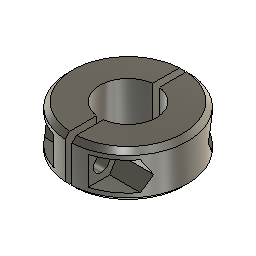
Dual Shaft Shredder (Autodesk Fusion 360 archive; units mm, degrees)
design "Double-Split Shaft Collars (20x20)"
Autodesk Fusion 360 part; units mm, degrees
sketch "Sketch1" plane through (0, 0, 0) normal (0, 0, 1) x (1, 0, 0)
  circle A0 centre (0, 0) radius 6
  circle A1 centre (0, 0) radius 13
  circle A2 centre (0, 0) radius 6.15
  line L0 (0.75, 20) -> (-0.75, 20)
  line L1 (-0.75, 20) -> (-0.75, -20)
  line L2 (-0.75, -20) -> (0.75, -20)
  line L3 (0.75, -20) -> (0.75, 20)
  line L4 (0.75, 20) -> (-0.75, -20) construction
  line L5 (-0.75, 20) -> (0.75, -20) construction
  line L6 (0.75, -9.336) -> (-0.75, -9.336)
  line L7 (0, -6.15) -> (0, -13)
  point P0 (0, -6.15)
  point P1 (0, -13)
  dimension "d1" = 12
  dimension "d2" = 0.15
  dimension "d5" = 1.5
  dimension "d7" = 26
  dimension "d44" = 3.186
  dimension "d45" = 40
  dimension "d46" = 6.85
  constraint coincident A0.centre A1.centre
  constraint concentric A0 A1
  constraint horizontal L0
  constraint perpendicular L0 L1
  constraint parallel L0 L2
  constraint parallel L1 L3
  constraint coincident L4 A0.centre
  constraint coincident L5 A0.centre
  constraint coincident L3 L6.start
  constraint coincident L1 L6.end
  constraint perpendicular L1 L6
  constraint coincident A2 P0
  constraint coincident A1 P1
  constraint coincident P0 L7.start
  constraint coincident P1 L7.end
  constraint parallel L3 L7
  measures "d1" diameter of A0
  measures "d5" distance of L1.end L2.end
  measures "d7" diameter of A1
  measures "d44" distance of L6 P0
  measures "d45" vertical distance of L0.end L2.end
  measures "d46" distance of P0 P1
extrude "Extrude1" add sketch "Sketch1" along normal blind 10 contours A1 A2 L3 | A1 A2 L1 makes body 1 at (8.6713, -9.6855, 6.6667) makes body 2 at (-7.1905, -10.8304, 3.3333)
sketch "Sketch2" plane through (-0.75, 0, 0) normal (1, 0, 0) x (0, 1, 0)
  line L0 (6.1041, 0) -> (12.9783, 0)
  line L1 (12.9783, 0) -> (12.9783, 10)
  line L2 (12.9783, 10) -> (6.1041, 10)
  line L3 (6.1041, 10) -> (6.1041, 0)
  line L4 (7.7514, 8.1) -> (5.9617, 5)
  line L5 (5.9617, 5) -> (7.7514, 1.9)
  line L6 (7.7514, 1.9) -> (11.331, 1.9)
  line L7 (11.331, 1.9) -> (13.1208, 5)
  line L8 (13.1208, 5) -> (11.331, 8.1)
  line L9 (11.331, 8.1) -> (7.7514, 8.1)
  circle A0 centre (9.5412, 5) radius 1.75
  line L10 (9.5412, 5) -> (6.1041, 5) construction
  line L11 (9.5412, 5) -> (12.9783, 5) construction
  line L12 (9.5412, 5) -> (9.5412, 0) construction
  line L13 (9.5412, 5) -> (9.5412, 10) construction
  line L14 (11.331, 8.1) -> (12.9783, 8.1)
  line L15 (11.331, 1.9) -> (12.9783, 1.9)
  line L16 (0, 0) -> (0, 10)
  line L17 (-9.5412, 5) -> (-9.5412, 10) construction
  line L18 (-12.9783, 0) -> (-12.9783, 10)
  line L19 (-9.5412, 5) -> (-12.9783, 5) construction
  line L20 (-11.331, 1.9) -> (-13.1208, 5)
  line L21 (-11.331, 8.1) -> (-12.9783, 8.1)
  line L22 (-7.7514, 1.9) -> (-11.331, 1.9)
  line L23 (-6.1041, 10) -> (-6.1041, 0)
  line L24 (-11.331, 1.9) -> (-12.9783, 1.9)
  circle A1 centre (-9.5412, 5) radius 1.75
  line L25 (-9.5412, 5) -> (-9.5412, 0) construction
  line L26 (-9.5412, 5) -> (-6.1041, 5) construction
  line L27 (-5.9617, 5) -> (-7.7514, 1.9)
  line L28 (-13.1208, 5) -> (-11.331, 8.1)
  line L29 (-11.331, 8.1) -> (-7.7514, 8.1)
  line L30 (-7.7514, 8.1) -> (-5.9617, 5)
  point P0 (9.5412, 5)
  point P1 (-9.5412, 5)
  dimension "d17" = 3.1
  dimension "d18" = 3.5
  constraint coincident P0 A0.centre
  constraint midpoint L3 L10.end
  constraint midpoint L1 L11.end
  constraint coincident L0 L12.end
  constraint perpendicular L0 L12
  constraint coincident L2 L13.end
  constraint perpendicular L2 L13
  constraint equal L10 L11
  constraint coincident L1 L14.end
  constraint perpendicular L1 L14
  constraint coincident L1 L15.end
  constraint perpendicular L1 L15
  constraint horizontal L10
  constraint coincident L16.start origin
  constraint vertical L16
  constraint horizontal L9
  constraint symmetric L0.start L16 L23.end
  constraint symmetric L0.end L16 L18.start
  constraint symmetric L1.end L16 L18.end
  constraint symmetric L2.end L16 L23.start
  constraint symmetric L4.start L16 L29.end
  constraint symmetric L4.end L16 L27.start
  constraint symmetric L5.end L16 L22.start
  constraint symmetric L6.end L16 L20.start
  constraint symmetric L7.end L16 L20.end
  constraint symmetric L8.end L16 L21.start
  constraint symmetric P0 L16 P1
  constraint symmetric A0 L16 A1
  constraint symmetric L10.end L16 L26.end
  constraint symmetric L11.end L16 L19.end
  constraint symmetric L12.end L16 L25.end
  constraint symmetric L13.end L16 L17.end
  constraint symmetric L14.end L16 L21.end
  constraint symmetric L15.end L16 L24.end
  measures "d17" distance of P0 L9
  measures "d18" diameter of A0
extrude "Extrude2" cut sketch "Sketch2" along normal mid plane 200 contours A0 | A1 bodies 1 2
extrude "Extrude3" cut sketch "Sketch2" against normal blind 10 from surface at -3 contours L3 L4 L5 | L1 L3 L4 L5 L6 L7 L8 L9 | L1 L7 L15 | L1 L8 L14 | A0 | L18 L20 L24 | L18 L20 L28 | L18 L20 L22 L23 L27 L28 L29 L30 | L18 L21 L28 | L23 L27 L30 | A1 bodies 2
extrude "Extrude4" cut sketch "Sketch2" along normal blind 100 from surface at 4.5 contours L3 L4 L5 | L1 L3 L4 L5 L6 L7 L8 L9 | L1 L7 L15 | L1 L8 L14 | L18 L20 L24 | L18 L20 L28 | L18 L20 L22 L23 L27 L28 L29 L30 | L18 L21 L28 | L23 L27 L30 | A1 bodies 1
chamfer "Chamfer1" distance 1 angle 45 4 edges at (13, 0, 0) (-13, 0, 0) (13, 0, 10) (-13, 0, 10) on bodies 1 2
ref_plane "WorkPlane1" through (0, -16, 0) normal (0, 1, 0) x (0, 0, 1)
sketch "Sketch3" plane through (0, -16, 0) normal (0, 1, 0) x (1, 0, 0)
  line L0 (2.7682, -5.085) -> (2.7681, -3.3241)
  spline S0 degree 5 poles (0.7027, -4.5337) (0.7103, -4.5353) (0.7255, -4.5381) (0.7483, -4.5414) (0.7791, -4.5438) (0.8177, -4.5436) (0.8566, -4.5399) (0.8955, -4.5325) (0.9341, -4.5209) (0.9719, -4.5044) (1.0082, -4.4824) (1.0425, -4.4542) (1.0739, -4.4193) (1.1016, -4.3775) (1.125, -4.3289) (1.1434, -4.274) (1.1562, -4.2138) (1.1629, -4.1493) (1.1634, -4.0822) (1.1577, -4.0144) (1.146, -3.9481) (1.1285, -3.8854) (1.1057, -3.8281) (1.0777, -3.7778) (1.0448, -3.7354) (1.0072, -3.7014) (0.9735, -3.681) (0.9462, -3.6696) (0.9271, -3.6638) (0.9173, -3.6613) knots 0 0 0 0 0 0 0.04 0.08 0.12 0.16 0.2 0.24 0.28 0.32 0.36 0.4 0.44 0.48 0.52 0.56 0.6 0.64 0.68 0.72 0.76 0.8 0.84 0.88 0.92 0.96 1 1 1 1 1 1
  line L1 (-3.1848, -3.0239) -> (-0.2225, -1.1432)
  arc A0 (0.0476, -6.9119) -> (-0.0024, -6.8619) centre (0.0476, -6.8619) cw
  line L2 (-1.3972, -3.7392) -> (-1.0488, -3.7773)
  line L3 (-1.627, -6.2849) -> (0.0512, -7.3504)
  line L4 (0.0476, -6.3678) -> (0.924, -6.3678)
  line L5 (1.6752, -6.3065) -> (0.8223, -5.3819)
  line L6 (3.2854, -7.1282) -> (0.0564, -9.2039)
  line L7 (-1.6303, -4.4396) -> (-1.102, -4.3813)
  line L8 (-0.0261, -5.4201) -> (-0.0261, -5.3437)
  line L9 (3.2854, -5.085) -> (3.2854, -7.1282)
  line L10 (0.0632, -3.9467) -> (0.0632, -4.4154)
  spline S1 degree 5 poles (1.7234, -4.437) (1.723, -4.4408) (1.722, -4.4487) (1.7198, -4.4614) (1.7155, -4.4798) (1.7078, -4.5055) (1.6978, -4.5337) (1.6855, -4.5642) (1.6713, -4.5965) (1.6556, -4.6296) (1.6392, -4.6624) (1.6226, -4.6937) (1.6066, -4.7223) (1.5916, -4.7474) (1.5781, -4.7684) (1.5661, -4.7851) (1.5578, -4.7951) (1.5523, -4.8006) (1.5489, -4.8035) (1.5473, -4.8047) knots 0 0 0 0 0 0 0.066667 0.133333 0.2 0.266667 0.333333 0.4 0.466667 0.533333 0.6 0.666667 0.733333 0.8 0.866667 0.933333 1 1 1 1 1 1
  line L11 (-1.0788, -5.1426) -> (-1.1684, -4.8048)
  line L12 (-2.6786, -5.0947) -> (-2.6686, -6.8612)
  line L13 (0.1369, -4.8048) -> (1.7234, -4.8047)
  line L14 (-2.6692, -3.3091) -> (0.0547, -1.5798)
  line L15 (-0.6159, -5.5515) -> (-1.0229, -5.5515)
  line L16 (-1.6325, -5.3094) -> (-1.2801, -6.5052)
  line L17 (0.1369, -4.8048) -> (-0.4862, -4.8048)
  line L18 (1.7234, -5.0851) -> (1.7234, -3.8946)
  line L19 (0.7027, -4.5337) -> (0.7027, -3.6651)
  line L20 (0.8223, -5.3819) -> (1.7234, -5.3819)
  line L21 (-1.6274, -3.8853) -> (0.0512, -2.8196)
  line L22 (3.2854, -5.085) -> (3.2853, -3.0418)
  line L23 (-3.1957, -5.0948) -> (-3.1848, -3.0239)
  line L24 (1.7234, -5.0851) -> (1.7234, -6.2754)
  line L25 (2.7682, -5.085) -> (2.7682, -6.8459)
  line L26 (-1.6338, -5.0945) -> (-1.627, -6.2849)
  line L27 (0.9173, -3.6613) -> (0.7027, -3.6651)
  line L28 (-0.6538, -6.9028) -> (-0.5276, -6.9028)
  line L29 (0.924, -6.3678) -> (-0.0261, -5.4201)
  line L30 (-0.2225, -1.1432) -> (0.0565, -0.9661)
  arc A1 (-0.0024, -6.4178) -> (0.0476, -6.3678) centre (0.0476, -6.4178) cw
  spline S2 degree 5 poles (-1.102, -4.3813) (-1.0994, -4.3879) (-1.094, -4.4007) (-1.0852, -4.4189) (-1.0722, -4.4412) (-1.0536, -4.4657) (-1.0329, -4.4869) (-1.0102, -4.505) (-0.9858, -4.5202) (-0.9601, -4.5327) (-0.9337, -4.543) (-0.9072, -4.5513) (-0.8808, -4.5579) (-0.8548, -4.5628) (-0.8291, -4.5657) (-0.8032, -4.5659) (-0.7769, -4.563) (-0.7501, -4.5564) (-0.7232, -4.546) (-0.6972, -4.532) (-0.6737, -4.5148) (-0.6542, -4.4953) (-0.6398, -4.4745) (-0.6311, -4.4533) (-0.6271, -4.4326) (-0.6266, -4.4132) (-0.6278, -4.3955) (-0.6292, -4.3796) (-0.6305, -4.365) (-0.6326, -4.3504) (-0.6371, -4.3345) (-0.6459, -4.3162) (-0.6606, -4.2952) (-0.6818, -4.2721) (-0.709, -4.2489) (-0.7408, -4.228) (-0.7756, -4.2116) (-0.8113, -4.2014) (-0.8463, -4.1978) (-0.8792, -4.1992) (-0.909, -4.2032) (-0.935, -4.2065) (-0.9567, -4.2059) (-0.9737, -4.1984) (-0.9858, -4.1823) (-0.993, -4.1564) (-0.9948, -4.1275) (-0.9938, -4.1011) (-0.9922, -4.0814) (-0.9911, -4.071) knots 0 0 0 0 0 0 0.022222 0.044444 0.066667 0.088889 0.111111 0.133333 0.155556 0.177778 0.2 0.222222 0.244444 0.266667 0.288889 0.311111 0.333333 0.355556 0.377778 0.4 0.422222 0.444444 0.466667 0.488889 0.511111 0.533333 0.555556 0.577778 0.6 0.622222 0.644444 0.666667 0.688889 0.711111 0.733333 0.755556 0.777778 0.8 0.822222 0.844444 0.866667 0.888889 0.911111 0.933333 0.955556 0.977778 1 1 1 1 1 1
  line L31 (-0.4893, -6.8744) -> (0.1369, -4.8048)
  line L32 (-1.1684, -4.8048) -> (-1.6322, -4.8024)
  line L33 (-3.1842, -7.1465) -> (0.0564, -9.2039)
  line L34 (-3.1957, -5.0948) -> (-3.1842, -7.1465)
  spline S3 degree 5 poles (-1.0488, -3.7773) (-1.0435, -3.768) (-1.0328, -3.75) (-1.0169, -3.7246) (-0.9961, -3.6939) (-0.9705, -3.6606) (-0.9455, -3.6323) (-0.921, -3.609) (-0.8972, -3.5902) (-0.874, -3.5754) (-0.8515, -3.564) (-0.8299, -3.5552) (-0.8091, -3.5484) (-0.7889, -3.543) (-0.7692, -3.539) (-0.7495, -3.5365) (-0.7293, -3.536) (-0.7084, -3.5381) (-0.6864, -3.5433) (-0.6638, -3.5517) (-0.641, -3.5634) (-0.6188, -3.5783) (-0.5981, -3.5958) (-0.5797, -3.6156) (-0.5642, -3.6371) (-0.5522, -3.6597) (-0.5437, -3.683) (-0.5388, -3.7065) (-0.5376, -3.7299) (-0.5398, -3.7531) (-0.5452, -3.7759) (-0.5537, -3.7985) (-0.5651, -3.8207) (-0.5794, -3.8423) (-0.5968, -3.8625) (-0.6177, -3.8805) (-0.6424, -3.8953) (-0.6709, -3.9061) (-0.703, -3.9124) (-0.7379, -3.9144) (-0.7745, -3.9129) (-0.8112, -3.9092) (-0.8463, -3.9046) (-0.8785, -3.9005) (-0.9065, -3.8982) (-0.9299, -3.8982) (-0.9484, -3.9012) (-0.9622, -3.9071) (-0.9719, -3.9159) (-0.9782, -3.9273) (-0.9818, -3.9409) (-0.9837, -3.9564) (-0.9846, -3.9734) (-0.9851, -3.9914) (-0.9858, -4.0103) (-0.987, -4.0299) (-0.9883, -4.046) (-0.9896, -4.0584) (-0.9906, -4.0668) (-0.9911, -4.071) knots 0 0 0 0 0 0 0.018182 0.036364 0.054545 0.072727 0.090909 0.109091 0.127273 0.145455 0.163636 0.181818 0.2 0.218182 0.236364 0.254545 0.272727 0.290909 0.309091 0.327273 0.345455 0.363636 0.381818 0.4 0.418182 0.436364 0.454545 0.472727 0.490909 0.509091 0.527273 0.545455 0.563636 0.581818 0.6 0.618182 0.636364 0.654545 0.672727 0.690909 0.709091 0.727273 0.745455 0.763636 0.781818 0.8 0.818182 0.836364 0.854545 0.872727 0.890909 0.909091 0.927273 0.945455 0.963636 0.981818 1 1 1 1 1 1
  line L35 (1.7234, -6.2754) -> (0.0512, -7.3504)
  line L36 (-0.5884, -5.1425) -> (-1.0788, -5.1426)
  line L37 (-0.0024, -6.8619) -> (-0.0024, -6.4178)
  line L38 (2.7681, -3.3241) -> (0.0547, -1.5798)
  line L39 (3.2853, -3.0418) -> (0.3344, -1.1447)
  line L40 (1.7234, -3.8946) -> (0.0512, -2.8196)
  line L41 (-1.0229, -5.5515) -> (-0.8136, -6.2122)
  line L42 (0.5197, -3.1208) -> (0.037, -3.1208)
  line L43 (-2.6686, -6.8612) -> (0.0547, -8.5903)
  arc A2 (-0.4893, -6.8744) -> (-0.5276, -6.9028) centre (-0.5276, -6.8628) cw
  line L44 (-0.8136, -6.2122) -> (-0.6159, -5.5515)
  line L45 (0.7334, -6.9119) -> (0.0476, -6.9119)
  spline S4 degree 5 poles (-0.1624, -4.0774) (-0.1492, -4.0711) (-0.1239, -4.0591) (-0.0895, -4.0426) (-0.0509, -4.024) (-0.0144, -4.006) (0.011, -3.9928) (0.0268, -3.9837) (0.0356, -3.9772) (0.0414, -3.9711) (0.0483, -3.9628) (0.0601, -3.9498) (0.0783, -3.9301) (0.1019, -3.9027) (0.1273, -3.8674) (0.1499, -3.8248) (0.1656, -3.7763) (0.1713, -3.7233) (0.1667, -3.6681) (0.1535, -3.6125) (0.1348, -3.5589) (0.1137, -3.5087) (0.0929, -3.4635) (0.0733, -3.4236) (0.054, -3.3889) (0.0332, -3.3585) (0.0084, -3.3317) (-0.0223, -3.3073) (-0.0597, -3.2848) (-0.1033, -3.264) (-0.1518, -3.2447) (-0.2034, -3.2271) (-0.2561, -3.2114) (-0.3084, -3.1979) (-0.3592, -3.1867) (-0.4078, -3.1778) (-0.4448, -3.1726) (-0.4714, -3.1697) (-0.4886, -3.1683) (-0.4971, -3.1677) knots 0 0 0 0 0 0 0.028571 0.057143 0.085714 0.114286 0.142857 0.171429 0.2 0.228571 0.257143 0.285714 0.314286 0.342857 0.371429 0.4 0.428571 0.457143 0.485714 0.514286 0.542857 0.571429 0.6 0.628571 0.657143 0.685714 0.714286 0.742857 0.771429 0.8 0.828571 0.857143 0.885714 0.914286 0.942857 0.971429 1 1 1 1 1 1
  line L46 (2.7682, -6.8459) -> (0.0547, -8.5903)
  line L47 (0.0565, -0.9661) -> (0.3344, -1.1447)
  line L48 (-1.6338, -5.0945) -> (-1.6274, -3.8853)
  spline S5 degree 5 poles (-1.6746, -4.5564) (-1.6709, -4.5624) (-1.6629, -4.5744) (-1.6495, -4.5925) (-1.6286, -4.6166) (-1.5972, -4.6469) (-1.5606, -4.6773) (-1.5183, -4.7076) (-1.4702, -4.7375) (-1.4155, -4.7669) (-1.3538, -4.7953) (-1.2849, -4.8222) (-1.2087, -4.847) (-1.126, -4.8691) (-1.0378, -4.8878) (-0.9462, -4.9022) (-0.853, -4.9117) (-0.7605, -4.9159) (-0.6708, -4.9147) (-0.5857, -4.9082) (-0.5062, -4.8971) (-0.4333, -4.8826) (-0.3669, -4.8657) (-0.3072, -4.8476) (-0.2535, -4.8291) (-0.2052, -4.8104) (-0.1614, -4.7908) (-0.1214, -4.7696) (-0.0844, -4.7456) (-0.0501, -4.7179) (-0.0187, -4.686) (0.009, -4.6503) (0.0322, -4.6112) (0.05, -4.5697) (0.0617, -4.5269) (0.0672, -4.4837) (0.067, -4.4409) (0.0618, -4.3993) (0.0526, -4.3595) (0.04, -4.3217) (0.0244, -4.286) (0.006, -4.2522) (-0.015, -4.2201) (-0.0388, -4.1894) (-0.0654, -4.1598) (-0.0947, -4.1313) (-0.1204, -4.1093) (-0.1409, -4.0932) (-0.1552, -4.0826) (-0.1624, -4.0774) knots 0 0 0 0 0 0 0.022222 0.044444 0.066667 0.088889 0.111111 0.133333 0.155556 0.177778 0.2 0.222222 0.244444 0.266667 0.288889 0.311111 0.333333 0.355556 0.377778 0.4 0.422222 0.444444 0.466667 0.488889 0.511111 0.533333 0.555556 0.577778 0.6 0.622222 0.644444 0.666667 0.688889 0.711111 0.733333 0.755556 0.777778 0.8 0.822222 0.844444 0.866667 0.888889 0.911111 0.933333 0.955556 0.977778 1 1 1 1 1 1
  line L49 (-2.6786, -5.0947) -> (-2.6692, -3.3091)
  line L50 (0.0527, -4.5564) -> (0.0527, -4.8048)
  line L51 (0.037, -3.1208) -> (0.037, -3.368)
  line L52 (-0.4862, -4.8048) -> (-0.5884, -5.1425)
  point P0 (-0.5387, -3.7178)
  point P1 (-0.5891, -3.606)
  point P2 (0.8856, -4.5337)
  point P3 (-0.9688, -3.9139)
  point P4 (1.1598, -4.1701)
  point P5 (-0.6883, -3.9089)
  point P6 (1.6852, -4.5643)
  point P7 (-0.9847, -3.9781)
  point P8 (1.6052, -4.7243)
  point P9 (-0.8774, -3.901)
  point P10 (1.0596, -4.4338)
  point P11 (1.1045, -3.83)
  point P12 (-0.5713, -3.8295)
  point P13 (0.1652, -3.7643)
  point P14 (0.0452, -5.2043)
  point P15 (0.1016, -3.4829)
  point P16 (-0.2437, -3.2154)
  point P17 (-0.0089, -3.3189)
  point P18 (-1.2016, -4.848)
  point P19 (-0.6447, -4.9119)
  point P20 (-1.5329, -4.6966)
  point P21 (-1.0059, -4.507)
  point P22 (-0.0631, -4.7275)
  point P23 (0.0527, -4.3635)
  point P24 (0.0527, -4.5564)
  point P25 (-0.0253, -4.2075)
  point P26 (-0.2617, -4.8316)
  point P27 (0.0252, -3.9843)
  point P28 (0.0652, -3.9443)
  point P29 (-0.9028, -3.5952)
  point P30 (-0.7946, -3.5447)
  point P31 (-0.6973, -3.5411)
  point P32 (-0.6389, -4.47)
  point P33 (-0.8754, -4.5587)
  point P34 (-0.8064, -4.204)
  point P35 (-0.7448, -4.5538)
  point P36 (-0.6291, -4.3813)
  point P37 (-0.6548, -4.3043)
  point P38 (-0.9548, -4.2043)
  constraint coincident L16.end L3
  constraint coincident L45.start L35
  constraint parallel L15 L45
  constraint perpendicular L37 L45
  constraint perpendicular L4 L37
  constraint coincident L8.end L31
  constraint parallel L8 L37
  constraint coincident L5.start L35
  constraint coincident L20.end L24
  constraint perpendicular L20 L24
  constraint coincident L13.end L18
  constraint perpendicular L13 L18
  constraint parallel L31 L52
  constraint coincident L32.end L48
  constraint perpendicular L32 L48
  constraint coincident L7.start L48
  constraint coincident S4.end L21
  constraint coincident L2.start L21
  constraint coincident L42.start L40
  constraint coincident L51.end S4
  constraint perpendicular L42 L51
  constraint coincident S1.start L18
  constraint coincident S1.end L13
  constraint coincident L16.start L26
  constraint coincident L10.start S4
  constraint coincident L10.end S5
  constraint tangent L31 A2
  constraint tangent L28 A2
  constraint tangent A0 L45
  constraint tangent A0 L37
  constraint tangent A1 L37
  constraint tangent L4 A1
  constraint parallel L1 L30
  constraint parallel L39 L47
  constraint coincident L50.end L17
  constraint perpendicular L17 L50
  constraint coincident P24 L50.start
emboss "Emboss1" [suppressed]
equation "d1 = Inner_Diameter"
equation "d7 = Outer_Diameter"
equation "d44 = d46 / 2.15"
equation "d45 = Inner_Diameter * 3.3333333333"
equation "d46 = ( Outer_Diameter - Inner_Diameter - 0.3 mm ) / 2"
equation "Inner_Diameter = 12 mm" comment "Edit Me!"
equation "Outer_Diameter = Inner_Diameter + 14 mm" comment "Do Not Change"

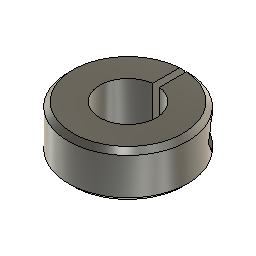
design "Shaft Collar (plastic)"
Autodesk Fusion 360 part; units mm, degrees
sketch "Sketch1" plane through (0, 0, 0) normal (0, 0, 1) x (1, 0, 0)
  circle A0 centre (0, 0) radius 6
  circle A1 centre (0, 0) radius 13
  circle A2 centre (0, 0) radius 6.15
  line L0 (0.75, 20) -> (-0.75, 20)
  line L1 (-0.75, 20) -> (-0.75, -20)
  line L2 (-0.75, -20) -> (0.75, -20)
  line L3 (0.75, -20) -> (0.75, 20)
  line L4 (0.75, 20) -> (-0.75, -20) construction
  line L5 (-0.75, 20) -> (0.75, -20) construction
  line L6 (0.75, -9.336) -> (-0.75, -9.336)
  line L7 (0, -6.15) -> (0, -13)
  point P0 (0, -6.15)
  point P1 (0, -13)
  dimension "d1" = 12
  dimension "d2" = 0.15
  dimension "d5" = 1.5
  dimension "d7" = 26
  dimension "d44" = 3.186
  dimension "d45" = 40
  dimension "d46" = 6.85
  constraint coincident A0.centre A1.centre
  constraint concentric A0 A1
  constraint horizontal L0
  constraint perpendicular L0 L1
  constraint parallel L0 L2
  constraint parallel L1 L3
  constraint coincident L4 A0.centre
  constraint coincident L5 A0.centre
  constraint coincident L3 L6.start
  constraint coincident L1 L6.end
  constraint perpendicular L1 L6
  constraint coincident A2 P0
  constraint coincident A1 P1
  constraint coincident P0 L7.start
  constraint coincident P1 L7.end
  constraint parallel L3 L7
  measures "d1" diameter of A0
  measures "d5" distance of L1.end L2.end
  measures "d7" diameter of A1
  measures "d44" distance of L6 P0
  measures "d45" vertical distance of L0.end L2.end
  measures "d46" distance of P0 P1
extrude "Extrude1" add sketch "Sketch1" along normal blind 10 contours A1 A2 L3 | A2 L3 L6 L7 | A1 A2 L1 | A2 L1 L6 L7 | A1 L3 L6 L7 | A1 L1 L6 L7
sketch "Sketch2" plane through (-0.75, 0, 0) normal (1, 0, 0) x (0, 1, 0)
  line L0 (6.1041, 0) -> (12.9783, 0)
  line L1 (12.9783, 0) -> (12.9783, 10)
  line L2 (12.9783, 10) -> (6.1041, 10)
  line L3 (6.1041, 10) -> (6.1041, 0)
  line L4 (7.637, 8.0311) -> (5.9641, 4.8665)
  line L5 (5.9641, 4.8665) -> (7.8683, 1.8354)
  line L6 (7.8683, 1.8354) -> (11.4454, 1.9689)
  line L7 (11.4454, 1.9689) -> (13.1183, 5.1335)
  line L8 (13.1183, 5.1335) -> (11.2141, 8.1646)
  line L9 (11.2141, 8.1646) -> (7.637, 8.0311)
  circle A0 centre (9.5412, 5) radius 1.75
  line L10 (9.5412, 5) -> (6.1041, 5) construction
  line L11 (9.5412, 5) -> (12.9783, 5) construction
  line L12 (9.5412, 5) -> (9.5412, 0) construction
  line L13 (9.5412, 5) -> (9.5412, 10) construction
  line L14 (11.2141, 8.1646) -> (12.9783, 8.1646)
  line L15 (11.4454, 1.9689) -> (12.9783, 1.9689)
  point P0 (9.5412, 5)
  dimension "d17" = 3.1
  dimension "d18" = 3.5
  constraint coincident P0 A0.centre
  constraint midpoint L3 L10.end
  constraint midpoint L1 L11.end
  constraint coincident L0 L12.end
  constraint perpendicular L0 L12
  constraint coincident L2 L13.end
  constraint perpendicular L2 L13
  constraint equal L10 L11
  constraint coincident L1 L14.end
  constraint perpendicular L1 L14
  constraint coincident L1 L15.end
  constraint perpendicular L1 L15
  constraint horizontal L10
  measures "d17" distance of P0 L9
  measures "d18" diameter of A0
extrude "Extrude2" cut sketch "Sketch2" along normal mid plane 200 contours A0
extrude "Extrude3" cut sketch "Sketch2" against normal blind 100 from surface at -3 contours L3 L4 L5 | L1 L3 L4 L5 L6 L7 L8 L9 | L1 L7 L15 | L1 L8 L14
extrude "Extrude4" cut sketch "Sketch2" along normal blind 100 from surface at 4.5 contours L3 L4 L5 | L1 L3 L4 L5 L6 L7 L8 L9 | L1 L7 L15 | L1 L8 L14
chamfer "Chamfer1" distance 1 angle 45 2 edges at (0, -13, 0) (0, -13, 10)
ref_plane "WorkPlane1" through (0, -16, 0) normal (0, 1, 0) x (0, 0, 1)
sketch "Sketch3" plane through (0, -16, 0) normal (0, 1, 0) x (1, 0, 0)
  line L0 (2.7682, -5.085) -> (2.7681, -3.3241)
  spline S0 degree 5 poles (0.7027, -4.5337) (0.7103, -4.5353) (0.7255, -4.5381) (0.7483, -4.5414) (0.7791, -4.5438) (0.8177, -4.5436) (0.8566, -4.5399) (0.8955, -4.5325) (0.9341, -4.5209) (0.9719, -4.5044) (1.0082, -4.4824) (1.0425, -4.4542) (1.0739, -4.4193) (1.1016, -4.3775) (1.125, -4.3289) (1.1434, -4.274) (1.1562, -4.2138) (1.1629, -4.1493) (1.1634, -4.0822) (1.1577, -4.0144) (1.146, -3.9481) (1.1285, -3.8854) (1.1057, -3.8281) (1.0777, -3.7778) (1.0448, -3.7354) (1.0072, -3.7014) (0.9735, -3.681) (0.9462, -3.6696) (0.9271, -3.6638) (0.9173, -3.6613) knots 0 0 0 0 0 0 0.04 0.08 0.12 0.16 0.2 0.24 0.28 0.32 0.36 0.4 0.44 0.48 0.52 0.56 0.6 0.64 0.68 0.72 0.76 0.8 0.84 0.88 0.92 0.96 1 1 1 1 1 1
  line L1 (-3.1848, -3.0239) -> (-0.2225, -1.1432)
  arc A0 (0.0476, -6.9119) -> (-0.0024, -6.8619) centre (0.0476, -6.8619) cw
  line L2 (-1.3972, -3.7392) -> (-1.0488, -3.7773)
  line L3 (-1.627, -6.2849) -> (0.0512, -7.3504)
  line L4 (0.0476, -6.3678) -> (0.924, -6.3678)
  line L5 (1.6752, -6.3065) -> (0.8223, -5.3819)
  line L6 (3.2854, -7.1282) -> (0.0564, -9.2039)
  line L7 (-1.6303, -4.4396) -> (-1.102, -4.3813)
  line L8 (-0.0261, -5.4201) -> (-0.0261, -5.3437)
  line L9 (3.2854, -5.085) -> (3.2854, -7.1282)
  line L10 (0.0632, -3.9467) -> (0.0632, -4.4154)
  spline S1 degree 5 poles (1.7234, -4.437) (1.723, -4.4408) (1.722, -4.4487) (1.7198, -4.4614) (1.7155, -4.4798) (1.7078, -4.5055) (1.6978, -4.5337) (1.6855, -4.5642) (1.6713, -4.5965) (1.6556, -4.6296) (1.6392, -4.6624) (1.6226, -4.6937) (1.6066, -4.7223) (1.5916, -4.7474) (1.5781, -4.7684) (1.5661, -4.7851) (1.5578, -4.7951) (1.5523, -4.8006) (1.5489, -4.8035) (1.5473, -4.8047) knots 0 0 0 0 0 0 0.066667 0.133333 0.2 0.266667 0.333333 0.4 0.466667 0.533333 0.6 0.666667 0.733333 0.8 0.866667 0.933333 1 1 1 1 1 1
  line L11 (-1.0788, -5.1426) -> (-1.1684, -4.8048)
  line L12 (-2.6786, -5.0947) -> (-2.6686, -6.8612)
  line L13 (0.1369, -4.8048) -> (1.7234, -4.8047)
  line L14 (-2.6692, -3.3091) -> (0.0547, -1.5798)
  line L15 (-0.6159, -5.5515) -> (-1.0229, -5.5515)
  line L16 (-1.6325, -5.3094) -> (-1.2801, -6.5052)
  line L17 (0.1369, -4.8048) -> (-0.4862, -4.8048)
  line L18 (1.7234, -5.0851) -> (1.7234, -3.8946)
  line L19 (0.7027, -4.5337) -> (0.7027, -3.6651)
  line L20 (0.8223, -5.3819) -> (1.7234, -5.3819)
  line L21 (-1.6274, -3.8853) -> (0.0512, -2.8196)
  line L22 (3.2854, -5.085) -> (3.2853, -3.0418)
  line L23 (-3.1957, -5.0948) -> (-3.1848, -3.0239)
  line L24 (1.7234, -5.0851) -> (1.7234, -6.2754)
  line L25 (2.7682, -5.085) -> (2.7682, -6.8459)
  line L26 (-1.6338, -5.0945) -> (-1.627, -6.2849)
  line L27 (0.9173, -3.6613) -> (0.7027, -3.6651)
  line L28 (-0.6538, -6.9028) -> (-0.5276, -6.9028)
  line L29 (0.924, -6.3678) -> (-0.0261, -5.4201)
  line L30 (-0.2225, -1.1432) -> (0.0565, -0.9661)
  arc A1 (-0.0024, -6.4178) -> (0.0476, -6.3678) centre (0.0476, -6.4178) cw
  spline S2 degree 5 poles (-1.102, -4.3813) (-1.0994, -4.3879) (-1.094, -4.4007) (-1.0852, -4.4189) (-1.0722, -4.4412) (-1.0536, -4.4657) (-1.0329, -4.4869) (-1.0102, -4.505) (-0.9858, -4.5202) (-0.9601, -4.5327) (-0.9337, -4.543) (-0.9072, -4.5513) (-0.8808, -4.5579) (-0.8548, -4.5628) (-0.8291, -4.5657) (-0.8032, -4.5659) (-0.7769, -4.563) (-0.7501, -4.5564) (-0.7232, -4.546) (-0.6972, -4.532) (-0.6737, -4.5148) (-0.6542, -4.4953) (-0.6398, -4.4745) (-0.6311, -4.4533) (-0.6271, -4.4326) (-0.6266, -4.4132) (-0.6278, -4.3955) (-0.6292, -4.3796) (-0.6305, -4.365) (-0.6326, -4.3504) (-0.6371, -4.3345) (-0.6459, -4.3162) (-0.6606, -4.2952) (-0.6818, -4.2721) (-0.709, -4.2489) (-0.7408, -4.228) (-0.7756, -4.2116) (-0.8113, -4.2014) (-0.8463, -4.1978) (-0.8792, -4.1992) (-0.909, -4.2032) (-0.935, -4.2065) (-0.9567, -4.2059) (-0.9737, -4.1984) (-0.9858, -4.1823) (-0.993, -4.1564) (-0.9948, -4.1275) (-0.9938, -4.1011) (-0.9922, -4.0814) (-0.9911, -4.071) knots 0 0 0 0 0 0 0.022222 0.044444 0.066667 0.088889 0.111111 0.133333 0.155556 0.177778 0.2 0.222222 0.244444 0.266667 0.288889 0.311111 0.333333 0.355556 0.377778 0.4 0.422222 0.444444 0.466667 0.488889 0.511111 0.533333 0.555556 0.577778 0.6 0.622222 0.644444 0.666667 0.688889 0.711111 0.733333 0.755556 0.777778 0.8 0.822222 0.844444 0.866667 0.888889 0.911111 0.933333 0.955556 0.977778 1 1 1 1 1 1
  line L31 (-0.4893, -6.8744) -> (0.1369, -4.8048)
  line L32 (-1.1684, -4.8048) -> (-1.6322, -4.8024)
  line L33 (-3.1842, -7.1465) -> (0.0564, -9.2039)
  line L34 (-3.1957, -5.0948) -> (-3.1842, -7.1465)
  spline S3 degree 5 poles (-1.0488, -3.7773) (-1.0435, -3.768) (-1.0328, -3.75) (-1.0169, -3.7246) (-0.9961, -3.6939) (-0.9705, -3.6606) (-0.9455, -3.6323) (-0.921, -3.609) (-0.8972, -3.5902) (-0.874, -3.5754) (-0.8515, -3.564) (-0.8299, -3.5552) (-0.8091, -3.5484) (-0.7889, -3.543) (-0.7692, -3.539) (-0.7495, -3.5365) (-0.7293, -3.536) (-0.7084, -3.5381) (-0.6864, -3.5433) (-0.6638, -3.5517) (-0.641, -3.5634) (-0.6188, -3.5783) (-0.5981, -3.5958) (-0.5797, -3.6156) (-0.5642, -3.6371) (-0.5522, -3.6597) (-0.5437, -3.683) (-0.5388, -3.7065) (-0.5376, -3.7299) (-0.5398, -3.7531) (-0.5452, -3.7759) (-0.5537, -3.7985) (-0.5651, -3.8207) (-0.5794, -3.8423) (-0.5968, -3.8625) (-0.6177, -3.8805) (-0.6424, -3.8953) (-0.6709, -3.9061) (-0.703, -3.9124) (-0.7379, -3.9144) (-0.7745, -3.9129) (-0.8112, -3.9092) (-0.8463, -3.9046) (-0.8785, -3.9005) (-0.9065, -3.8982) (-0.9299, -3.8982) (-0.9484, -3.9012) (-0.9622, -3.9071) (-0.9719, -3.9159) (-0.9782, -3.9273) (-0.9818, -3.9409) (-0.9837, -3.9564) (-0.9846, -3.9734) (-0.9851, -3.9914) (-0.9858, -4.0103) (-0.987, -4.0299) (-0.9883, -4.046) (-0.9896, -4.0584) (-0.9906, -4.0668) (-0.9911, -4.071) knots 0 0 0 0 0 0 0.018182 0.036364 0.054545 0.072727 0.090909 0.109091 0.127273 0.145455 0.163636 0.181818 0.2 0.218182 0.236364 0.254545 0.272727 0.290909 0.309091 0.327273 0.345455 0.363636 0.381818 0.4 0.418182 0.436364 0.454545 0.472727 0.490909 0.509091 0.527273 0.545455 0.563636 0.581818 0.6 0.618182 0.636364 0.654545 0.672727 0.690909 0.709091 0.727273 0.745455 0.763636 0.781818 0.8 0.818182 0.836364 0.854545 0.872727 0.890909 0.909091 0.927273 0.945455 0.963636 0.981818 1 1 1 1 1 1
  line L35 (1.7234, -6.2754) -> (0.0512, -7.3504)
  line L36 (-0.5884, -5.1425) -> (-1.0788, -5.1426)
  line L37 (-0.0024, -6.8619) -> (-0.0024, -6.4178)
  line L38 (2.7681, -3.3241) -> (0.0547, -1.5798)
  line L39 (3.2853, -3.0418) -> (0.3344, -1.1447)
  line L40 (1.7234, -3.8946) -> (0.0512, -2.8196)
  line L41 (-1.0229, -5.5515) -> (-0.8136, -6.2122)
  line L42 (0.5197, -3.1208) -> (0.037, -3.1208)
  line L43 (-2.6686, -6.8612) -> (0.0547, -8.5903)
  arc A2 (-0.4893, -6.8744) -> (-0.5276, -6.9028) centre (-0.5276, -6.8628) cw
  line L44 (-0.8136, -6.2122) -> (-0.6159, -5.5515)
  line L45 (0.7334, -6.9119) -> (0.0476, -6.9119)
  spline S4 degree 5 poles (-0.1624, -4.0774) (-0.1492, -4.0711) (-0.1239, -4.0591) (-0.0895, -4.0426) (-0.0509, -4.024) (-0.0144, -4.006) (0.011, -3.9928) (0.0268, -3.9837) (0.0356, -3.9772) (0.0414, -3.9711) (0.0483, -3.9628) (0.0601, -3.9498) (0.0783, -3.9301) (0.1019, -3.9027) (0.1273, -3.8674) (0.1499, -3.8248) (0.1656, -3.7763) (0.1713, -3.7233) (0.1667, -3.6681) (0.1535, -3.6125) (0.1348, -3.5589) (0.1137, -3.5087) (0.0929, -3.4635) (0.0733, -3.4236) (0.054, -3.3889) (0.0332, -3.3585) (0.0084, -3.3317) (-0.0223, -3.3073) (-0.0597, -3.2848) (-0.1033, -3.264) (-0.1518, -3.2447) (-0.2034, -3.2271) (-0.2561, -3.2114) (-0.3084, -3.1979) (-0.3592, -3.1867) (-0.4078, -3.1778) (-0.4448, -3.1726) (-0.4714, -3.1697) (-0.4886, -3.1683) (-0.4971, -3.1677) knots 0 0 0 0 0 0 0.028571 0.057143 0.085714 0.114286 0.142857 0.171429 0.2 0.228571 0.257143 0.285714 0.314286 0.342857 0.371429 0.4 0.428571 0.457143 0.485714 0.514286 0.542857 0.571429 0.6 0.628571 0.657143 0.685714 0.714286 0.742857 0.771429 0.8 0.828571 0.857143 0.885714 0.914286 0.942857 0.971429 1 1 1 1 1 1
  line L46 (2.7682, -6.8459) -> (0.0547, -8.5903)
  line L47 (0.0565, -0.9661) -> (0.3344, -1.1447)
  line L48 (-1.6338, -5.0945) -> (-1.6274, -3.8853)
  spline S5 degree 5 poles (-1.6746, -4.5564) (-1.6709, -4.5624) (-1.6629, -4.5744) (-1.6495, -4.5925) (-1.6286, -4.6166) (-1.5972, -4.6469) (-1.5606, -4.6773) (-1.5183, -4.7076) (-1.4702, -4.7375) (-1.4155, -4.7669) (-1.3538, -4.7953) (-1.2849, -4.8222) (-1.2087, -4.847) (-1.126, -4.8691) (-1.0378, -4.8878) (-0.9462, -4.9022) (-0.853, -4.9117) (-0.7605, -4.9159) (-0.6708, -4.9147) (-0.5857, -4.9082) (-0.5062, -4.8971) (-0.4333, -4.8826) (-0.3669, -4.8657) (-0.3072, -4.8476) (-0.2535, -4.8291) (-0.2052, -4.8104) (-0.1614, -4.7908) (-0.1214, -4.7696) (-0.0844, -4.7456) (-0.0501, -4.7179) (-0.0187, -4.686) (0.009, -4.6503) (0.0322, -4.6112) (0.05, -4.5697) (0.0617, -4.5269) (0.0672, -4.4837) (0.067, -4.4409) (0.0618, -4.3993) (0.0526, -4.3595) (0.04, -4.3217) (0.0244, -4.286) (0.006, -4.2522) (-0.015, -4.2201) (-0.0388, -4.1894) (-0.0654, -4.1598) (-0.0947, -4.1313) (-0.1204, -4.1093) (-0.1409, -4.0932) (-0.1552, -4.0826) (-0.1624, -4.0774) knots 0 0 0 0 0 0 0.022222 0.044444 0.066667 0.088889 0.111111 0.133333 0.155556 0.177778 0.2 0.222222 0.244444 0.266667 0.288889 0.311111 0.333333 0.355556 0.377778 0.4 0.422222 0.444444 0.466667 0.488889 0.511111 0.533333 0.555556 0.577778 0.6 0.622222 0.644444 0.666667 0.688889 0.711111 0.733333 0.755556 0.777778 0.8 0.822222 0.844444 0.866667 0.888889 0.911111 0.933333 0.955556 0.977778 1 1 1 1 1 1
  line L49 (-2.6786, -5.0947) -> (-2.6692, -3.3091)
  line L50 (0.0527, -4.5564) -> (0.0527, -4.8048)
  line L51 (0.037, -3.1208) -> (0.037, -3.368)
  line L52 (-0.4862, -4.8048) -> (-0.5884, -5.1425)
  point P0 (-0.5387, -3.7178)
  point P1 (-0.5891, -3.606)
  point P2 (0.8856, -4.5337)
  point P3 (-0.9688, -3.9139)
  point P4 (1.1598, -4.1701)
  point P5 (-0.6883, -3.9089)
  point P6 (1.6852, -4.5643)
  point P7 (-0.9847, -3.9781)
  point P8 (1.6052, -4.7243)
  point P9 (-0.8774, -3.901)
  point P10 (1.0596, -4.4338)
  point P11 (1.1045, -3.83)
  point P12 (-0.5713, -3.8295)
  point P13 (0.1652, -3.7643)
  point P14 (0.0452, -5.2043)
  point P15 (0.1016, -3.4829)
  point P16 (-0.2437, -3.2154)
  point P17 (-0.0089, -3.3189)
  point P18 (-1.2016, -4.848)
  point P19 (-0.6447, -4.9119)
  point P20 (-1.5329, -4.6966)
  point P21 (-1.0059, -4.507)
  point P22 (-0.0631, -4.7275)
  point P23 (0.0527, -4.3635)
  point P24 (0.0527, -4.5564)
  point P25 (-0.0253, -4.2075)
  point P26 (-0.2617, -4.8316)
  point P27 (0.0252, -3.9843)
  point P28 (0.0652, -3.9443)
  point P29 (-0.9028, -3.5952)
  point P30 (-0.7946, -3.5447)
  point P31 (-0.6973, -3.5411)
  point P32 (-0.6389, -4.47)
  point P33 (-0.8754, -4.5587)
  point P34 (-0.8064, -4.204)
  point P35 (-0.7448, -4.5538)
  point P36 (-0.6291, -4.3813)
  point P37 (-0.6548, -4.3043)
  point P38 (-0.9548, -4.2043)
  constraint coincident L16.end L3
  constraint coincident L45.start L35
  constraint parallel L15 L45
  constraint perpendicular L37 L45
  constraint perpendicular L4 L37
  constraint coincident L8.end L31
  constraint parallel L8 L37
  constraint coincident L5.start L35
  constraint coincident L20.end L24
  constraint perpendicular L20 L24
  constraint coincident L13.end L18
  constraint perpendicular L13 L18
  constraint parallel L31 L52
  constraint coincident L32.end L48
  constraint perpendicular L32 L48
  constraint coincident L7.start L48
  constraint coincident S4.end L21
  constraint coincident L2.start L21
  constraint coincident L42.start L40
  constraint coincident L51.end S4
  constraint perpendicular L42 L51
  constraint coincident S1.start L18
  constraint coincident S1.end L13
  constraint coincident L16.start L26
  constraint coincident L10.start S4
  constraint coincident L10.end S5
  constraint tangent L31 A2
  constraint tangent L28 A2
  constraint tangent A0 L45
  constraint tangent A0 L37
  constraint tangent A1 L37
  constraint tangent L4 A1
  constraint parallel L1 L30
  constraint parallel L39 L47
  constraint coincident L50.end L17
  constraint perpendicular L17 L50
  constraint coincident P24 L50.start
emboss "Emboss1" [rolled back] depth 0.5 horizontal distance 0 vertical distance 0 rotation angle 0
equation "d1 = Inner_Diameter"
equation "d7 = Outer_Diameter"
equation "d44 = d46 / 2.15"
equation "d45 = Inner_Diameter * 3.3333333333"
equation "d46 = ( Outer_Diameter - Inner_Diameter - 0.3 mm ) / 2"
equation "Inner_Diameter = 12 mm" comment "Edit Me!"
equation "Outer_Diameter = Inner_Diameter + 14 mm" comment "Do Not Change"
